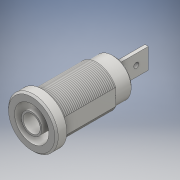
# Autodesk Inventor part: Prise banane
Saved by Autodesk Inventor 2016 SP1 (Build 200210100, 210)
## iProperties
Created: 2018-06-13
Part Number: Prise banane
Material: Plastique ABS
Document SubType Name: Modeling
Designer: dimercur
Density: 1.06 g/cm^3
Appearance: Lisse - Blanc
Author: dimercur
Autodesk Inventor part; units mm, degrees
ref_plane "YZ Plane" through (0, 0, 0) normal (1, 0, 0) x (0, 1, 0)
ref_plane "XZ Plane" through (0, 0, 0) normal (0, 1, 0) x (-1, 0, 0)
ref_plane "XY Plane" through (0, 0, 0) normal (0, 0, 1) x (1, 0, 0)
sketch "Esquisse1" plane through (0, 0, 0) normal (0, 1, 0) x (-1, 0, 0)
  circle A0 centre (0, 0) radius 7.25
  dimension "d0" = 14.5
  constraints: 1 centre point, 1 coincident
  measures "d0" diameter of A0
extrude "Extrusion1" add sketch "Esquisse1" along normal blind 3
sketch "Esquisse2" plane through (0, 3, 0) normal (0, 1, 0) x (1, 0, 0)
  circle A0 centre (0, 0) radius 6
  dimension "d3" = 12
  constraints: 1 centre point, 1 coincident
  measures "d3" diameter of A0
extrude "Extrusion2" add sketch "Esquisse2" along normal blind 16
sketch "Esquisse3" plane through (0, 19, 0) normal (0, 1, 0) x (1, 0, 0)
  circle A0 centre (0, 0) radius 5.5
  dimension "d6" = 11
  constraints: 1 centre point, 1 coincident
  measures "d6" diameter of A0
extrude "Extrusion3" add sketch "Esquisse3" along normal blind 5
thread "Filetage1" size "M12x0.5" class "6g" standard "ANSI Metric M Profile" full length
sketch "Esquisse4" plane through (0, 24, 0) normal (0, 1, 0) x (1, 0, 0)
  line L0 (-7.5, 3) -> (-5.5, 3)
  line L1 (-5.5, 3) -> (-5.5, -3)
  line L2 (-5.5, -3) -> (-7.5, -3)
  line L3 (-7.5, -3) -> (-7.5, 3)
  line L4 (7.5, 3) -> (5.5, 3)
  line L5 (5.5, 3) -> (5.5, -3)
  line L6 (5.5, -3) -> (7.5, -3)
  line L7 (7.5, -3) -> (7.5, 3)
  circle A0 centre (0, 0) radius 5.5 projected
  circle A1 centre (0, 0) radius 5.5 projected
  point P0 (-5.5, 0)
  point P1 (5.5, 0)
  dimension "d11" = 2
  dimension "d12" = 11
  dimension "d13" = 5.5
  dimension "d14" = 5.5
  dimension "d15" = 11
  dimension "d16" = 2
  dimension "d17" = 6
  dimension "d18" = 3
  constraints: 16 end point, 4 parallel, 4 point on circle, 2 horizontal, 2 perpendicular, 2 point on line
  measures "d11" distance of L0.start L0.end
  measures "d12" distance of A0.end A0.start
  measures "d13" distance of point (0, 0) A0.start
  measures "d14" distance from line of point (0, 0) L1
  measures "d15" distance between parallel lines of L1 L5
  measures "d16" distance of L4.start L4.end
  measures "d17" distance from line of L6.end L4
  measures "d18" vertical distance of A0.start L0.start
extrude "Extrusion4" cut sketch "Esquisse4" against normal blind 21 contours L5 L4 L7 L6 | L0 L1 L2 L3
sketch "Esquisse5" plane through (0, 24, 0) normal (0, 1, 0) x (1, 0, 0)
  line L0 (-0.5, 3) -> (0.5, 3)
  line L1 (0.5, 3) -> (0.5, -3)
  line L2 (0.5, -3) -> (-0.5, -3)
  line L3 (-0.5, -3) -> (-0.5, 3)
  point P0 (0, 0)
  dimension "d21" = 1
  dimension "d22" = 0.5
  dimension "d23" = 6
  dimension "d24" = 3
  constraints: 8 end point, 2 parallel, 1 horizontal, 1 perpendicular
  measures "d21" distance of L0.start L0.end
  measures "d22" horizontal distance of point (0, 0) L0.start
  measures "d23" distance between parallel lines of L2 L0
  measures "d24" vertical distance of L0.start point (0, 0)
extrude "Extrusion5" add sketch "Esquisse5" along normal blind 10
sketch "Esquisse6" plane through (0, 0, 0) normal (0, -1, 0) x (1, 0, 0)
  circle A0 centre (0, 0) radius 5
  circle A1 centre (0, 0) radius 3
  circle A2 centre (0, 0) radius 2.5
  dimension "d27" = 10
  dimension "d28" = 6
  dimension "d29" = 5
  constraints: 3 centre point, 3 coincident
  measures "d27" diameter of A0
  measures "d28" diameter of A1
  measures "d29" diameter of A2
extrude "Extrusion6" cut sketch "Esquisse6" against normal blind 10
chamfer "Chanfrein1" distance 0.5 angle 45 6 edges at (7.25, 0, 0) (-5.5, 24, 0) (0, 34, -3) (0, 34, 3) (0.5, 34, 0) (-0.5, 34, 0)
sketch "Esquisse7" plane through (0.5, 24, 3) normal (1, 0, 0) x (0, 0, -1)
  circle A0 centre (3, 6) radius 0.75
  line L0 (-2, 0) -> (8, 0) projected
  point P0 (3, -24)
  dimension "d35" = 1.5
  dimension "d36" = 6
  constraints: 1 centre point
  measures "d35" diameter of A0
  measures "d36" distance from line of L0 A0.centre
extrude "Extrusion7" cut sketch "Esquisse7" against normal blind 10
equation "\"d14\" = d13"
equation "\"d15\" = d12"
equation "\"d16\" = d11"
equation "\"d18\" = 0.5 * d17"
equation "\"d22\" = 0.5 * d21"
equation "\"d24\" = 0.5 * d23"
